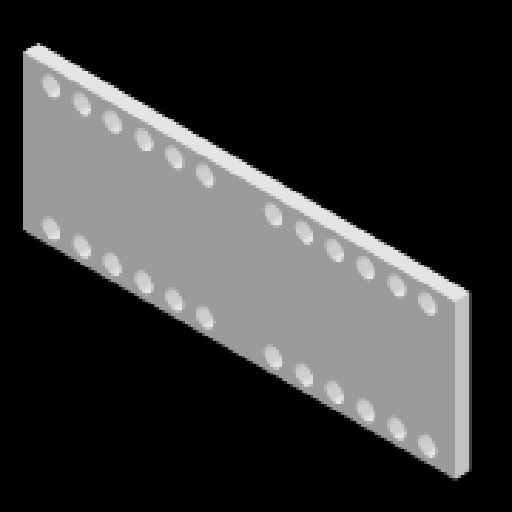
# Autodesk Inventor part: CombineTestBase
Saved by Autodesk Inventor 2025 (Build 290162000, 162)
## iProperties
Created: 2025-01-20
Part Number: CombineTestBase
Material: Generic
Document SubType Name: Modeling
Designer: Trevor
Density: 1 g/cm^3
Appearance: Default
Author: Trevor
Autodesk Inventor part; units mm, degrees
ref_plane "YZ Plane" through (0, 0, 0) normal (1, 0, 0) x (0, 1, 0)
ref_plane "XZ Plane" through (0, 0, 0) normal (0, 1, 0) x (-1, 0, 0)
ref_plane "XY Plane" through (0, 0, 0) normal (0, 0, 1) x (1, 0, 0)
sketch "Sketch1" plane through (0, 0, 0) normal (0, 0, 1) x (1, 0, 0)
  line L0 (65, 8) -> (65, -5) projected
  line L1 (-5, -5) -> (-5, 8) projected
  line L2 (-5, 8) -> (65, 8) projected
  line L3 (65, 8) -> (65, -5) projected
  line L4 (65, -5) -> (-5, -5) projected
  line L5 (-5, 15) -> (65, 15)
  line L6 (65, 15) -> (65, -10)
  line L7 (65, -10) -> (-5, -10)
  line L8 (-5, -10) -> (-5, 15)
  line L9 (-5, 15) -> (65, -10) construction
  line L10 (65, 15) -> (-5, -10) construction
  point P0 (0, 0)
  point P1 (30, 2.5)
  dimension "d0" = 25
  constraints: 12 end point, 2 midpoint, 2 parallel, 1 perpendicular
  measures "d0" distance of L5.end L6.end
extrude "Extrusion1" add sketch "Sketch1" along normal blind 2.5
sketch "Sketch2" plane through (0, 0, 0) normal (0, 0, -1) x (-1, 0, 0)
  line L0 (-60, 0) -> (0, 0) projected
  line L1 (0, 0) -> (0, 3) projected
  line L2 (-60, 3) -> (0, 3) projected
  line L3 (-60, 0) -> (-60, 3) projected
  line L4 (0.2, -0.2) -> (-60.2, -0.2)
  line L5 (-60.2, -0.2) -> (-60.2, 3.2)
  line L6 (-60.2, 3.2) -> (0.2, 3.2)
  line L7 (0.2, 3.2) -> (0.2, -0.2)
  line L8 (-61.2, -1.2) -> (1.2, -1.2)
  line L9 (1.2, -1.2) -> (1.2, 4.2)
  line L10 (1.2, 4.2) -> (-61.2, 4.2)
  line L11 (-61.2, 4.2) -> (-61.2, -1.2)
  dimension "d3" = 0.2
  dimension "d4" = 1
  constraints: 16 end point, 6 other
  measures "d3" distance between parallel lines of L0 L4
  measures "d4" distance between parallel lines of L4 L8
extrude "Extrusion2" add sketch "Sketch2" along normal blind 3 contours L11 L10 L9 L8
fillet "Fillet1" radius 2 4 edges at (30, -1.2, 0) (-1.2, 1.5, 0) (30, 4.2, 0) (61.2, 1.5, 0)
sketch "Sketch3" plane through (0, 0, 0) normal (0, 0, -1) x (-1, 0, 0)
  line L0 (-65, -10.0193) -> (-65, -5)
  line L1 (-65, -10) -> (-65, 15) projected
  line L2 (-65, -7.5097) -> (5, -7.5097) construction
  line L3 (5, 15) -> (5, -10) projected
  line L4 (-47.2, 0) -> (-43.8, 0) projected
  line L5 (-45.5, 0) -> (-45.5, -10) construction
  circle A0 centre (-45.5, -7.5097) radius 1.5
  line L6 (-16.2, 0) -> (-12.8, 0) projected
  line L7 (-14.5, 0) -> (-14.5, -7.5097)
  circle A1 centre (-14.5, -7.5097) radius 1.5
  circle A2 centre (-50.5, -7.5097) radius 1.5
  circle A3 centre (-55.5, -7.5097) radius 1.5
  circle A4 centre (-60.5, -7.5097) radius 1.5
  line L8 (5, -10) -> (-65, -10) construction
  line L9 (-30, -10) -> (-30, 15) construction
  circle A5 centre (-40.5, -7.5097) radius 1.5
  circle A6 centre (-35.5, -7.5097) radius 1.5
  circle A7 centre (-14.5, -7.5097) radius 1.5
  circle A8 centre (-9.5, -7.5097) radius 1.5
  circle A9 centre (-4.5, -7.5097) radius 1.5
  circle A10 centre (0.5, -7.5097) radius 1.5
  circle A11 centre (-19.5, -7.5097) radius 1.5
  circle A12 centre (-24.5, -7.5097) radius 1.5
  line L10 (-65, 2.5) -> (5, 2.5) construction
  line L11 (-65, 12.5097) -> (5, 12.5097) construction
  circle A13 centre (-45.5, 12.5097) radius 1.5
  circle A14 centre (-14.5, 12.5097) radius 1.5
  circle A15 centre (-50.5, 12.5097) radius 1.5
  circle A16 centre (-55.5, 12.5097) radius 1.5
  circle A17 centre (-60.5, 12.5097) radius 1.5
  circle A18 centre (-40.5, 12.5097) radius 1.5
  circle A19 centre (-35.5, 12.5097) radius 1.5
  circle A20 centre (0.5, 12.5097) radius 1.5
  circle A21 centre (-4.5, 12.5097) radius 1.5
  circle A22 centre (-9.5, 12.5097) radius 1.5
  circle A23 centre (-19.5, 12.5097) radius 1.5
  circle A24 centre (-24.5, 12.5097) radius 1.5
  point P0 (0, 0)
  dimension "d10" = 3
  dimension "d11" = 3
  dimension "d14" = 5
  dimension "d21" = 5
  constraints: 25 centre point, 19 symmetric about line, 14 end point, 6 midpoint, 5 point on line, 2 horizontal, 2 perpendicular, 2 vertical, 1 coincident, 1 collinear, 28 other
  measures "d10" diameter of A0
  measures "d11" diameter of A1
  measures "d14" distance of A0.centre A2.centre
  measures "d21" distance of A0.centre A5.centre
extrude "Extrusion3" cut sketch "Sketch3" against normal up to surface (2.5 mm away)
equation "\"d26\" = d21"
body "Solid1"
